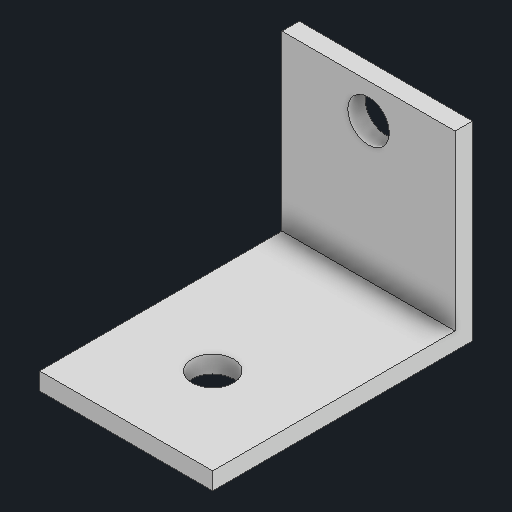
# Autodesk Inventor part: Teste Suporte
Saved by Autodesk Inventor 2026.2 (Build 302298010, 298A)
## iProperties
Created: 2025-11-09
Part Number: Teste Suporte
Material: Genérico
Document SubType Name: Modeling
Designer: Rubens
Density: 1 g/cm^3
Appearance: Padrão
Author: Rubens
Autodesk Inventor part; units mm, degrees
ref_plane "YZ Plane" through (0, 0, 0) normal (1, 0, 0) x (0, 1, 0)
ref_plane "XZ Plane" through (0, 0, 0) normal (0, 1, 0) x (-1, 0, 0)
ref_plane "XY Plane" through (0, 0, 0) normal (0, 0, 1) x (1, 0, 0)
sketch "Esboço1" plane through (0, 0, 0) normal (0, 0, 1) x (1, 0, 0)
  line L0 (0, 0) -> (50, 0)
  line L1 (50, 0) -> (50, 55)
  line L2 (50, 55) -> (0, 55)
  line L3 (0, 55) -> (0, 0)
  circle A0 centre (25, 45) radius 6
  dimension "d0" = 50
  dimension "d1" = 55
  dimension "d2" = 12
  dimension "d8" = 45
  dimension "d14" = 25
  constraints: 8 end point, 2 parallel, 1 centre point, 1 horizontal, 1 perpendicular
  measures "d0" distance of L2.end L1.end
  measures "d1" distance of L1.end L0.end
  measures "d2" diameter of A0
  measures "d8" distance from line of L0 A0.centre
  measures "d14" distance from line of L1 A0.centre
extrude "Extrusão1" add sketch "Esboço1" along normal blind 5
sketch "Esboço2" plane through (0, 0, 5) normal (0, 0, 1) x (1, 0, 0)
  line L0 (50, 0) -> (50, 55) projected
  line L1 (0, 0) -> (50, 0)
  line L2 (50, 0) -> (50, 5)
  line L3 (50, 5) -> (0, 5)
  line L4 (0, 5) -> (0, 0)
  dimension "d5" = 5
  constraints: 8 end point, 2 parallel, 1 horizontal, 1 perpendicular, 1 point on line
  measures "d5" distance of L2.end L1.end
extrude "Extrusão2" add sketch "Esboço2" along normal blind 70
sketch "Esboço3" plane through (0, 5, 5) normal (0, 1, 0) x (1, 0, 0)
  circle A0 centre (25, -45) radius 6
  line L0 (50, -70) -> (0, -70) projected
  line L1 (50, 0) -> (50, -70) projected
  point P0 (0, 5)
  dimension "d9" = 12
  dimension "d10" = 25
  dimension "d11" = 25
  constraints: 1 centre point
  measures "d9" diameter of A0
  measures "d10" distance from line of L0 A0.centre
  measures "d11" distance from line of L1 A0.centre
extrude "Extrusão3" cut sketch "Esboço3" against normal blind 40
